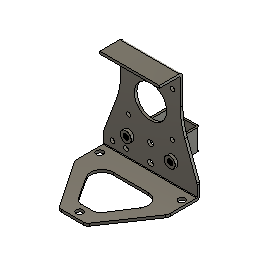
Top Tower mount v5 (Autodesk Fusion 360 design; units mm, degrees)
Autodesk Fusion 360 part; units mm, degrees
sketch "Sketch1" plane through (0, 0, 0) normal (0, 1, 0) x (1, 0, 0)
  line L0 (0, 0) -> (66, 0)
  line L1 (0, -22.45) -> (0, 0)
  line L2 (33, 0) -> (33, -56.9)
  line L3 (33, -56.9) -> (40.9149, -56.9)
  line L4 (33, -56.9) -> (25.0851, -56.9)
  line L5 (43.3932, -55.5906) -> (66, -22.45)
  line L6 (22.6068, -55.5906) -> (0, -22.45)
  arc A0 (40.9149, -56.9) -> (43.3932, -55.5906) centre (40.9149, -53.9) ccw
  arc A1 (22.6068, -55.5906) -> (25.0851, -56.9) centre (25.0851, -53.9) ccw
  line L7 (0, 0) -> (66, 0)
  line L8 (66, 0) -> (66, -1.86)
  line L9 (66, -1.86) -> (0, -1.86)
  line L10 (0, -1.86) -> (0, 0)
  line L11 (0, 0) -> (66, 0)
  line L12 (0, -15.9) -> (0, 0)
  line L13 (33, -56.9) -> (33, -46.75)
  line L14 (33, -46.75) -> (40, -46.75)
  line L15 (33, -46.75) -> (26, -46.75)
  line L16 (33, -15.9) -> (6, -15.9)
  line L17 (11.5053, -24.3919) -> (26, -46.75)
  line L18 (33, -15.9) -> (49.8797, -15.9)
  line L19 (40, -46.75) -> (54.4947, -24.3919)
  line L20 (66, 0) -> (66, -1.86)
  line L21 (66, 0) -> (66, -6.3)
  line L22 (66, 0) -> (66, -22.45)
  line L23 (66, -6.3) -> (66, -8.7)
  line L24 (66, -8.7) -> (64.4, -8.7)
  line L25 (64.4, -8.7) -> (62, -8.7)
  circle A2 centre (62, -8.7) radius 2.4
  circle A3 centre (4, -8.7) radius 2.4
  line L26 (33, -56.9) -> (33, -54.3)
  line L27 (33, -54.3) -> (33, -51.9)
  circle A4 centre (33, -51.9) radius 2.4
  line L28 (49.8797, -15.9) -> (60, -15.9)
  line L29 (54.4947, -24.3919) -> (60, -15.9)
  line L30 (11.5053, -24.3919) -> (6, -15.9)
  line L31 (33, -1.86, 0) -> (33, -1.86, 71.95)
  point P0 (42.5, -56.9)
  point P1 (23.5, -56.9)
  point P2 (60, -15.9)
  dimension "d1" = 66
  dimension "d2" = 22.45
  dimension "d3" = 56.9
  dimension "d4" = 9.5
  dimension "d5" = 9.5
  dimension "d6" = 3
  dimension "d7" = 1.86
  dimension "d9" = 15.9
  dimension "d10" = 10.15
  dimension "d11" = 7
  dimension "d12" = 7
  dimension "d14" = 27
  dimension "d17" = 6.3
  dimension "d18" = 2.4
  dimension "d19" = 1.6
  dimension "d20" = 2.4
  dimension "d21" = 2.6
  dimension "d22" = 2.4
  dimension "d29" = 71.95
  constraint horizontal L0
  constraint vertical L1
  constraint coincident L0.start L1.end
  constraint midpoint L0 L2.start
  constraint perpendicular L0 L2
  constraint perpendicular L2 L3
  constraint perpendicular L2 L4
  constraint coincident P0 L3
  constraint coincident P0 L5
  constraint tangent L3 A0
  constraint tangent L5 A0
  constraint coincident P1 L4
  constraint coincident P1 L6
  constraint tangent L4 A1
  constraint tangent L6 A1
  constraint equal A0 A1
  constraint horizontal L7
  constraint vertical L8
  constraint horizontal L9
  constraint vertical L10
  constraint horizontal L11
  constraint vertical L12
  constraint perpendicular L4 L13
  constraint perpendicular L13 L14
  constraint perpendicular L2 L15
  constraint perpendicular L2 L16
  constraint perpendicular L2 L18
  constraint coincident P2 L18
  constraint coincident P2 L19
  constraint perpendicular L9 L20
  constraint perpendicular L9 L21
  constraint perpendicular L7 L22
  constraint parallel L21 L23
  constraint perpendicular L22 L24
  constraint parallel L24 L25
  constraint coincident L25.end A2.centre
  constraint coincident L24.end A2
  constraint symmetric L2 A2 A3
  constraint perpendicular L4 L26
  constraint perpendicular L14 L27
  constraint coincident L27.end A4.centre
  constraint coincident L26.end A4
  constraint parallel L18 L28
  constraint coincident P2 L28.end
  constraint parallel L19 L29
  constraint parallel L17 L30
  measures "d1" distance of L0.start L0.end
  measures "d2" distance of L0.start L1.start
  measures "d3" distance of L2.start L2.end
  measures "d4" distance of L2.end P0
  measures "d5" distance of L2.end P1
  measures "d6" radius of A0
  measures "d7" distance of L0.start L9.end
  measures "d9" distance of L0.start L12.start
  measures "d10" distance of L2.end L13.end
  measures "d11" distance of L13.end L14.end
  measures "d12" distance of L13.end L15.end
  measures "d14" distance of L16.start P2
  measures "d17" distance of L0.end L21.end
  measures "d18" distance of L21.end L23.end
  measures "d19" distance of L23.end L24.end
  measures "d20" distance of L24.end L25.end
  measures "d21" distance of L2.end L26.end
  measures "d22" distance of L26.end L27.end
extrude "Extrude1" add sketch "Sketch1" along normal blind 1.83 contours L1 L2 L4 L6 A1 L9 L12 L13 L15 L16 L17 L26 A4 L30 | L2 L3 L5 A0 L9 L13 L14 L18 L19 L21 L22 L23 L26 A4 L28 L29 makes body 1
fillet "Fillet1" radius 8 2 edges at (6, 0.915, 15.9) (60, 0.915, 15.9) on bodies 1
fillet "Fillet2" radius 5 4 edges at (66, 0.915, 22.45) (0, 0.915, 22.45) (40, 0.915, 46.75) (26, 0.915, 46.75) on bodies 1
sketch "Sketch2" plane through (0, 0, 1.86) normal (0, 0, -1) x (-1, 0, 0)
  line L0 (-66, 0) -> (0, 0)
  line L1 (0, 0) -> (0, 1.83)
  line L2 (0, 1.83) -> (-66, 1.83)
  line L3 (-66, 1.83) -> (-66, 0)
  circle A0 centre (-33, 44.05) radius 11.45
  circle A1 centre (-48.5, 59.55) radius 1.5
  circle A2 centre (-17.5, 59.55) radius 1.5
  circle A3 centre (-17.5, 28.55) radius 1.5
  circle A4 centre (-48.5, 28.55) radius 1.5
  line L4 (-33, 0) -> (-33, 4.82)
  line L5 (-33, 4.82) -> (-33, 6.82)
  circle A5 centre (-33, 6.82) radius 2
  line L6 (-33, 8.82) -> (-33, 16.62)
  line L7 (-33, 16.62) -> (-33, 18.62)
  circle A6 centre (-33, 18.62) radius 2
  line L8 (-33, 71.95) -> (-54, 71.95)
  line L9 (-33, 71.95) -> (-12, 71.95)
  line L10 (-12, 71.95) -> (-54, 71.95)
  line L11 (-54, 71.95) -> (-54, 70.15)
  line L12 (-54, 70.15) -> (-12, 70.15)
  line L13 (-12, 70.15) -> (-12, 71.95)
  line L14 (-31, 6.82) -> (-17.3, 6.82)
  line L15 (-17.3, 6.82) -> (-15.65, 6.82)
  circle A7 centre (-15.65, 6.82) radius 1.65
  line L16 (-14, 6.82) -> (-8, 6.82)
  line L17 (-8, 6.82) -> (-7.7363, 6.82)
  line L18 (-7.7363, 6.82) -> (-6.0863, 6.82)
  circle A8 centre (-6.0863, 6.82) radius 1.65
  line L19 (-33, 0) -> (-33, 15.8)
  line L20 (-33, 15.8) -> (-19, 15.8)
  line L21 (-33, 15.8) -> (-47, 15.8)
  line L22 (-19, 15.8) -> (-17.44, 15.8)
  circle A9 centre (-17.44, 15.8) radius 1.56
  line L23 (-47, 15.8) -> (-48.56, 15.8)
  circle A10 centre (-48.56, 15.8) radius 1.56
  circle A11 centre (-48.56, 15.8) radius 3.9
  circle A12 centre (-17.44, 15.8) radius 3.9
  line L24 (-66, 0) -> (0, 0)
  line L25 (0, 0) -> (0, 9.3139)
  line L26 (-66, 9.3139) -> (-66, 0)
  line L27 (-54, 70.15) -> (-12, 70.15)
  line L28 (-12, 70.15) -> (-12, 57.15)
  line L29 (-54, 57.15) -> (-54, 70.15)
  line L30 (-54, 57.15) -> (-12, 57.15)
  line L31 (-12, 57.15) -> (-12, 51.1771)
  line L32 (-54, 51.1771) -> (-54, 57.15)
  line L33 (-65.7601, 10.6427) -> (-57.1567, 33.6928)
  arc A13 (-57.1567, 33.6928) -> (-54, 51.1771) centre (-104, 51.1771) ccw
  arc A14 (-12, 51.1771) -> (-8.8433, 33.6928) centre (38, 51.1771) ccw
  line L34 (-0.2399, 10.6427) -> (-8.8433, 33.6928)
  arc A15 (0, 9.3139) -> (-0.2399, 10.6427) centre (-3.8, 9.3139) ccw
  arc A16 (-65.7601, 10.6427) -> (-66, 9.3139) centre (-62.2, 9.3139) ccw
  point P0 (-33, 0)
  point P1 (-33, 44.05)
  point P2 (-33, 71.95)
  point P3 (-66, 10)
  point P4 (-54, 42.15)
  dimension "d32" = 31
  dimension "d33" = 31
  dimension "d34" = 3
  dimension "d35" = 3
  dimension "d36" = 3
  dimension "d37" = 3
  dimension "d38" = 4.82
  dimension "d39" = 2
  dimension "d40" = 7.8
  dimension "d41" = 2
  dimension "d42" = 21
  dimension "d43" = 21
  dimension "d44" = 1.8
  dimension "d45" = 13.7
  dimension "d46" = 1.65
  dimension "d47" = 6
  dimension "d48" = 1.65
  dimension "d49" = 15.8
  dimension "d50" = 14
  dimension "d51" = 14
  dimension "d52" = 1.56
  dimension "d53" = 1.56
  dimension "d54" = 7.8
  dimension "d55" = 7.8
  dimension "d56" = 10
  dimension "d57" = 13
  dimension "d58" = 15
  dimension "d59" = 50
  dimension "d60" = 3.8
  constraint coincident P1 A0.centre
  constraint coincident P0 L4.start
  constraint perpendicular L0 L4
  constraint coincident L5.end A5.centre
  constraint coincident L4.end A5
  constraint coincident A5 L6.start
  constraint vertical L6
  constraint parallel L6 L7
  constraint coincident L7.end A6.centre
  constraint coincident L6.end A6
  constraint coincident P2 L8.start
  constraint horizontal L9
  constraint horizontal L10
  constraint vertical L11
  constraint horizontal L12
  constraint vertical L13
  constraint coincident A5 L14.start
  constraint perpendicular L5 L14
  constraint parallel L14 L15
  constraint coincident L15.end A7.centre
  constraint coincident L14.end A7
  constraint coincident A7 L16.start
  constraint parallel L15 L16
  constraint parallel L16 L18
  constraint coincident L18.end A8.centre
  constraint coincident L17.end A8
  constraint parallel L4 L19
  constraint perpendicular L6 L20
  constraint perpendicular L6 L21
  constraint perpendicular L7 L22
  constraint coincident L22.end A9.centre
  constraint coincident L20.end A9
  constraint parallel L21 L23
  constraint coincident L23.end A10.centre
  constraint coincident L21.end A10
  constraint concentric A10 A11
  constraint concentric A9 A12
  constraint horizontal L24
  constraint vertical L25
  constraint vertical L26
  constraint coincident L0.start L3.end
  constraint horizontal L27
  constraint vertical L28
  constraint vertical L29
  constraint horizontal L30
  constraint vertical L31
  constraint vertical L32
  constraint coincident P4 L32
  constraint coincident P4 L33
  constraint tangent L32 A13
  constraint tangent L33 A13
  constraint symmetric L19 L32.start L31.end
  constraint symmetric L19 L33.end A14.end
  constraint symmetric L19 A13 A14
  constraint tangent L34 A15
  constraint tangent L25 A15
  constraint coincident P3 L26
  constraint coincident P3 L33
  constraint tangent L26 A16
  constraint tangent L33 A16
  constraint equal A15 A16
  measures "d32" distance of A1.centre A2.centre
  measures "d33" distance of A1.centre A4.centre
  measures "d34" diameter of A1
  measures "d35" diameter of A2
  measures "d36" diameter of A3
  measures "d37" diameter of A4
  measures "d38" distance of P0 L4.end
  measures "d39" distance of L4.end L5.end
  measures "d40" distance of L6.start L6.end
  measures "d41" distance of L6.end L7.end
  measures "d42" distance of P2 L8.end
  measures "d43" distance of P2 L9.end
  measures "d44" distance of L9.end L12.end
  measures "d45" distance of L14.start L14.end
  measures "d46" distance of L14.end L15.end
  measures "d47" distance of L16.start L16.end
  measures "d48" distance of L17.end L18.end
  measures "d49" distance of P0 L19.end
  measures "d50" distance of L19.end L20.end
  measures "d51" distance of L19.end L21.end
  measures "d52" distance of L20.end L22.end
  measures "d53" distance of L21.end L23.end
  measures "d54" diameter of A11
  measures "d55" diameter of A12
  measures "d56" distance of L0.start P3
  measures "d57" distance of L11.end L29.start
  measures "d58" distance of L29.start P4
  measures "d59" radius of A13
  measures "d60" radius of A15
extrude "Extrude2" add sketch "Sketch2" along normal blind 1.83 contours L0 L2 L3 L4 L19 L24 L26 | L0 L1 L2 L4 L19 L24 L25 | L2 L25 L26 L30 L31 L32 L33 A13 A14 L34 A15 A16 | L12 L27 L28 L29 L30 | L8 L9 L10 L11 L12 L13 L27 | A11 | A12 bodies 1
extrude "Extrude3" add sketch "Sketch2" against normal blind 14.8 contours L8 L9 L10 L11 L12 L13 L27 bodies 1
fillet "Fillet3" radius 2.5 2 edges at (33, 71.95, 0.03) (33, 0, 0.03) on bodies 1
fillet "Fillet4" radius 0.4 2 edges at (33, 70.15, 1.86) (33, 1.83, 1.86) on bodies 1
extrude "Extrude4" add sketch "Sketch2" against normal blind 2 contours A11 | A12 bodies 1
fillet "Fillet5" radius 0.05 2 edges at (52.1961, 17.2103, 3.86) (21.0761, 17.2103, 3.86) on bodies 1
thread "Thread1" "ISO Metric profile 4.0 M4x0.7 6H" major diameter 4.1095 minor diameter 3.332 pitch 0.7 angle 60 modelled right hand crest width 0.193 on face at (15.8878, 15.9553, 1.3067) crest through (15.774, 15.8, 3.685) on face at (47.0078, 15.6447, 1.3067) crest through (46.894, 15.8, 3.685) on bodies 1
sketch "Sketch3" plane through (0, 0, 0.03) normal (0, 0, -1) x (-1, 0, 0)
  spline S0 degree 3 poles (-18.3161, 13.9414) (-18.5414, 14.0746) (-18.739, 14.2499) (-19.0486, 14.6596) (-19.1605, 14.8879) (-19.2864, 15.3656) (-19.3026, 15.6095) (-19.2401, 16.08) (-19.1657, 16.3025) (-18.9814, 16.6232) (-18.8991, 16.7339) (-18.712, 16.9305) (-18.6086, 17.0162) (-18.4959, 17.0886) knots 0 0 0 0 0.078521 0.078521 0.154183 0.154183 0.226983 0.226983 0.296921 0.296921 0.338304 0.338304 0.378622 0.378622 0.378622 0.378622
  arc A0 (-15.9986, 16.6354) -> (-18.4959, 17.0886) centre (-17.44, 15.8) ccw
  spline S1 degree 3 poles (-15.9986, 16.6354) (-15.867, 16.4589) (-15.7719, 16.2579) (-15.6599, 15.8218) (-15.6476, 15.5899) (-15.7122, 15.1247) (-15.792, 14.8962) (-16.0381, 14.4734) (-16.2051, 14.285) (-16.5286, 14.0368) (-16.6653, 13.9561) (-16.9581, 13.8272) (-17.1135, 13.7802) (-17.2728, 13.7521) knots 0 0 0 0 0.066052 0.066052 0.134957 0.134957 0.206715 0.206715 0.281323 0.281323 0.328596 0.328596 0.376941 0.376941 0.376941 0.376941
  arc A1 (-18.3161, 13.9414) -> (-17.2728, 13.7521) centre (-17.44, 15.8) ccw
  spline S2 degree 3 poles (-49.4361, 13.9414) (-49.6614, 14.0746) (-49.859, 14.2499) (-50.1686, 14.6596) (-50.2805, 14.8879) (-50.4064, 15.3656) (-50.4226, 15.6095) (-50.3601, 16.08) (-50.2857, 16.3025) (-50.1014, 16.6232) (-50.0191, 16.7339) (-49.832, 16.9305) (-49.7286, 17.0162) (-49.6159, 17.0886) knots 0 0 0 0 0.078521 0.078521 0.154183 0.154183 0.226983 0.226983 0.296921 0.296921 0.338304 0.338304 0.378622 0.378622 0.378622 0.378622
  arc A2 (-47.1186, 16.6354) -> (-49.6159, 17.0886) centre (-48.56, 15.8) ccw
  spline S3 degree 3 poles (-47.1186, 16.6354) (-46.987, 16.4589) (-46.8919, 16.2579) (-46.7799, 15.8218) (-46.7676, 15.5899) (-46.8322, 15.1247) (-46.912, 14.8962) (-47.1581, 14.4734) (-47.3251, 14.285) (-47.6486, 14.0368) (-47.7853, 13.9561) (-48.0781, 13.8272) (-48.2335, 13.7802) (-48.3928, 13.7521) knots 0 0 0 0 0.066052 0.066052 0.134957 0.134957 0.206715 0.206715 0.281323 0.281323 0.328596 0.328596 0.376941 0.376941 0.376941 0.376941
  arc A3 (-49.4361, 13.9414) -> (-48.3928, 13.7521) centre (-48.56, 15.8) ccw
  line L0 (-66, 2.5) -> (0, 2.5)
  line L1 (0, 2.5) -> (0, 9.3139)
  arc A4 (0, 9.3139) -> (-0.2399, 10.6427) centre (-3.8, 9.3139) ccw
  line L2 (-0.2399, 10.6427) -> (-8.8433, 33.6928)
  arc A5 (-12, 51.1771) -> (-8.8433, 33.6928) centre (38, 51.1771) ccw
  line L3 (-12, 51.1771) -> (-12, 57.15)
  line L4 (-12, 57.15) -> (-12, 69.45)
  line L5 (-12, 69.45) -> (-54, 69.45)
  line L6 (-54, 69.45) -> (-54, 51.1771)
  arc A6 (-57.1567, 33.6928) -> (-54, 51.1771) centre (-104, 51.1771) ccw
  line L7 (-57.1567, 33.6928) -> (-65.7601, 10.6427)
  arc A7 (-65.7601, 10.6427) -> (-66, 9.3139) centre (-62.2, 9.3139) ccw
  line L8 (-66, 9.3139) -> (-66, 2.5)
  circle A8 centre (-33, 18.62) radius 2
  circle A9 centre (-15.65, 6.82) radius 1.65
  circle A10 centre (-17.5, 59.55) radius 1.5
  circle A11 centre (-48.5, 59.55) radius 1.5
  circle A12 centre (-33, 44.05) radius 11.45
  circle A13 centre (-6.0863, 6.82) radius 1.65
  circle A14 centre (-17.5, 28.55) radius 1.5
  circle A15 centre (-33, 6.82) radius 2
  circle A16 centre (-48.5, 28.55) radius 1.5
  line L9 (-48.56, 15.8) -> (-17.44, 15.8)
  line L10 (-48.56, 8.35) -> (-17.44, 8.35)
  arc A17 (-17.44, 8.35) -> (-17.44, 23.25) centre (-17.44, 15.8) ccw
  line L11 (-17.44, 23.25) -> (-48.56, 23.25)
  arc A18 (-48.56, 23.25) -> (-48.56, 8.35) centre (-48.56, 15.8) ccw
  line L12 (-48.56, 15.8) -> (-17.44, 15.8) construction
  circle A19 centre (-17.44, 15.8) radius 2.3
  circle A20 centre (-48.56, 15.8) radius 2.3
  line L13 (-22.84, 8.35) -> (-43.16, 8.35)
  line L14 (-43.16, 8.35) -> (-43.16, 23.25)
  line L15 (-43.16, 23.25) -> (-22.84, 23.25)
  line L16 (-22.84, 23.25) -> (-22.84, 8.35)
  line L17 (-22.84, 8.35) -> (-43.16, 23.25) construction
  line L18 (-43.16, 8.35) -> (-22.84, 23.25) construction
  line L19 (-22.84, 23.25) -> (-21.44, 23.25)
  line L20 (-21.44, 23.25) -> (-21.44, 8.35)
  line L21 (-21.44, 8.35) -> (-22.84, 8.35)
  line L22 (-22.84, 8.35) -> (-22.84, 23.25)
  line L23 (-43.16, 23.25) -> (-44.56, 23.25)
  line L24 (-44.56, 23.25) -> (-44.56, 8.35)
  line L25 (-44.56, 8.35) -> (-43.16, 8.35)
  line L26 (-43.16, 8.35) -> (-43.16, 23.25)
  line L27 (-21.44, 23.25) -> (-19.44, 23.25)
  line L28 (-19.44, 23.25) -> (-16.94, 23.25)
  line L29 (-2.94, 9.25) -> (-2.94, 6.75)
  line L30 (-5.44, 4.25) -> (-16.94, 4.25)
  line L31 (-19.44, 6.75) -> (-19.44, 23.25)
  circle A21 centre (-15.65, 6.82) radius 1
  circle A22 centre (-6.0863, 6.82) radius 1
  arc A23 (-2.94, 9.25) -> (-16.94, 23.25) centre (-16.94, 9.25) ccw
  arc A24 (-5.44, 4.25) -> (-2.94, 6.75) centre (-5.44, 6.75) ccw
  arc A25 (-19.44, 6.75) -> (-16.94, 4.25) centre (-16.94, 6.75) ccw
  point P0 (-33, 15.8)
  point P1 (-2.94, 23.25)
  point P2 (-19.44, 4.25)
  dimension "d73" = 14.9
  dimension "d74" = 4.6
  dimension "d75" = 4.6
  dimension "d76" = 20.32
  dimension "d77" = 1.4
  dimension "d78" = 1.4
  dimension "d89" = 2
  dimension "d90" = 16.5
  dimension "d91" = 19
  dimension "d92" = 2
  dimension "d93" = 2
  dimension "d94" = 14
  dimension "d95" = 2.5
  constraint coincident A2.centre A3.centre
  constraint coincident A0.centre A1.centre
  constraint tangent L10 A17
  constraint tangent A17 L11
  constraint parallel L10 L11
  constraint tangent L11 A18
  constraint tangent L10 A18
  constraint parallel L9 L12
  constraint concentric A0 A19
  constraint concentric A2 A20
  constraint horizontal L13
  constraint perpendicular L13 L14
  constraint parallel L13 L15
  constraint parallel L14 L16
  constraint coincident L10 L13.start
  constraint coincident L17 P0
  constraint coincident L18 P0
  constraint midpoint L9 P0
  constraint horizontal L19
  constraint vertical L20
  constraint horizontal L21
  constraint vertical L22
  constraint horizontal L23
  constraint vertical L24
  constraint horizontal L25
  constraint vertical L26
  constraint perpendicular L20 L27
  constraint horizontal L28
  constraint vertical L29
  constraint horizontal L30
  constraint vertical L31
  constraint concentric A9 A21
  constraint concentric A13 A22
  constraint coincident P1 L28
  constraint coincident P1 L29
  constraint tangent L28 A23
  constraint tangent L29 A23
  constraint tangent L29 A24
  constraint tangent L30 A24
  constraint coincident P2 L30
  constraint coincident P2 L31
  constraint tangent L30 A25
  constraint tangent L31 A25
  constraint equal A24 A25
  measures "d73" diameter of A17
  measures "d74" diameter of A19
  measures "d75" diameter of A20
  measures "d76" distance of L14.end L15.end
  measures "d77" distance of L15.end L19.end
  measures "d78" distance of L14.end L23.end
  measures "d89" distance of L19.end L27.end
  measures "d90" distance of L27.end P1
  measures "d91" distance of L27.end P2
  measures "d92" diameter of A21
  measures "d93" diameter of A22
  measures "d94" radius of A23
  measures "d95" radius of A24
extrude "Extrude5" add sketch "Sketch3" along normal blind 1.4 separate body contours L9 L10 A19 L20 L31 | L10 L11 A18 L24 | L10 A17 L11 A19 L28 L31 | L10 A17 L28 L29 L30 L31 A23 A24 A25 | L9 L11 A19 L20 L27 L31 makes body 2 at (46.9466, 10.1197, 0.03) makes body 3 at (9.1053, 13.3967, 0.03)
extrude "Extrude6" add sketch "Sketch3" along normal blind 21.4 contours A8 | A15 L10 L13 | A15 L9 L10 L13 L14 L16 L22 L26 | L9 L10 L16 L20 L21 L22 | L9 L10 L14 L24 L25 L26 | L9 L11 L16 L19 L20 L22 | L9 L11 L14 L15 L16 L22 L26 | L9 L11 L14 L23 L24 L26 picked at (-33, 8.5067) bodies 2 3
extrude "Extrude7" cut sketch "Sketch3" along normal blind 20.2 contours A8 | A15 L10 L13 | A15 L9 L10 L13 L14 L16 L22 L26 | L9 L11 L14 L15 L16 L22 L26 picked at (-33, 8.5067) bodies 2
fillet "Fillet6" radius 1.5 4 edges at (44.56, 15.8, -21.37) (21.44, 15.8, -21.37) (22.84, 15.8, 0.03) (43.16, 15.8, 0.03) on bodies 2
fillet "Fillet7" radius 0.2 4 edges at (22.84, 15.8, -20.17) (43.16, 15.8, -20.17) (44.56, 15.8, -1.37) (21.44, 15.8, -1.37) on bodies 2
thread "Thread2" "ISO Metric profile 2.0 M2x0.4 6H" major diameter 2.074 minor diameter 1.623 pitch 0.4 angle 60 modelled right hand crest width 0.1065 on face at (14.0021, 6.7378, -0.9033) crest through (14.8385, 6.82, -0.07) on face at (4.4383, 6.7378, -0.9033) crest through (5.2748, 6.82, -0.07) on bodies 2
